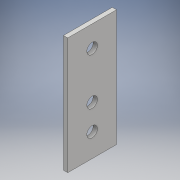
# Autodesk Inventor part: Mounting_wall
Saved by Autodesk Inventor 2017 (Build 210142000, 142)
## iProperties
Created: 2017-11-15
Part Number: Mounting_wall
Material: Generic
Document SubType Name: Modeling
Designer: julie
Density: 1 g/cm^3
Appearance: Default
Author: julie
Autodesk Inventor part; units mm, degrees
ref_plane "YZ Plane" through (0, 0, 0) normal (1, 0, 0) x (0, 1, 0)
ref_plane "XZ Plane" through (0, 0, 0) normal (0, 1, 0) x (-1, 0, 0)
ref_plane "XY Plane" through (0, 0, 0) normal (0, 0, 1) x (1, 0, 0)
sketch "Sketch1" plane through (0, 0, 0) normal (1, 0, 0) x (0, 1, 0)
  line L0 (0, 0) -> (23, 0)
  line L1 (23, 0) -> (23, -55)
  line L2 (23, -55) -> (0, -55)
  line L3 (0, -10) -> (0, -10)
  line L4 (0, -10) -> (0, -25)
  line L5 (0, -25) -> (0, -25)
  line L6 (0, -45) -> (0, -45)
  line L7 (0, -45) -> (0, -30)
  line L8 (0, -30) -> (0, -30)
  line L9 (0, -10) -> (0, 0)
  line L10 (0, -55) -> (0, -45)
  line L11 (0, -30) -> (0, -25)
  dimension "d0" = 23
  dimension "d1" = 55
  dimension "d2" = 0
  dimension "d3" = 15
  dimension "d4" = 10
  dimension "d5" = 15
  dimension "d6" = 10
  dimension "d10" = 0
  dimension "d11" = 0
  dimension "d12" = 0
  constraints: 24 end point, 9 perpendicular, 4 parallel, 3 horizontal
  measures "d0" distance of L1.end L2.end
  measures "d1" distance of L0.end L1.end
  measures "d2" distance of L3.start L3.end
  measures "d3" distance of L3.end L4.end
  measures "d4" distance from line of L0.start L3
  measures "d5" distance of L6.end L7.end
  measures "d6" distance between parallel lines of L2 L6
  measures "d10" distance of L6.start L6.end
  measures "d11" distance from line of L0.start L11
  measures "d12" distance of L7.end L8.end
extrude "Extrusion1" add sketch "Sketch1" along normal blind 2
sketch "Sketch3" plane through (2, 0, 0) normal (1, 0, 0) x (0, 0, -1)
  circle A0 centre (10, 11.5) radius 2.5
  circle A1 centre (32, 11.5) radius 2.5
  circle A2 centre (44, 11.5) radius 2.5
  line L0 (0, 23) -> (0, 0) projected
  line L1 (55, 23) -> (0, 23) projected
  dimension "d18" = 5
  dimension "d19" = 5
  dimension "d20" = 5
  dimension "d21" = 10
  dimension "d22" = 11.5
  dimension "d23" = 11.5
  dimension "d24" = 22
  dimension "d25" = 11.5
  dimension "d26" = 12
  constraints: 3 centre point
  measures "d18" diameter of A0
  measures "d19" diameter of A1
  measures "d20" diameter of A2
  measures "d21" distance from line of L0 A0.centre
  measures "d22" distance from line of L1 A0.centre
  measures "d23" distance from line of L1 A1.centre
  measures "d24" distance of A0.centre A1.centre
  measures "d25" distance from line of L1 A2.centre
  measures "d26" distance of A1.centre A2.centre
extrude "Extrusion3" cut sketch "Sketch3" against normal blind 10
body "Solid1"
